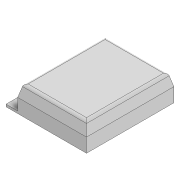
# Autodesk Inventor part: おもり
Saved by Autodesk Inventor 2020 (Build 240168000, 168)
## iProperties
Created: 2020-04-18
Part Number: おもり
Material: 一般
Document SubType Name: Modeling
Designer: highs
Density: 1 g/cm^3
Appearance: 既定
Author: highs
Autodesk Inventor part; units mm, degrees
ref_plane "YZ Plane" through (0, 0, 0) normal (1, 0, 0) x (0, 1, 0)
ref_plane "XZ Plane" through (0, 0, 0) normal (0, 1, 0) x (-1, 0, 0)
ref_plane "XY Plane" through (0, 0, 0) normal (0, 0, 1) x (1, 0, 0)
sketch "スケッチ1" plane through (0, 0, 0) normal (0, 0, 1) x (1, 0, 0)
  line L0 (0, 0) -> (138, 0)
  line L1 (138, 0) -> (138, 44)
  line L2 (138, 44) -> (20, 44)
  line L3 (20, 44) -> (20, 4)
  line L4 (20, 4) -> (0, 4)
  line L5 (0, 4) -> (0, 0)
  dimension "d0" = 20
  dimension "d1" = 4
  dimension "d2" = 40
  dimension "d3" = 118
  constraints: 12 end point, 4 perpendicular, 1 horizontal, 1 parallel
  measures "d0" distance of L3.end L4.end
  measures "d1" distance of L4.end L0.start
  measures "d2" distance of L2.end L3.end
  measures "d3" distance of L1.end L2.end
extrude "押し出し1" add sketch "スケッチ1" along normal blind 150
chamfer "面取り1" distance 5 distance2 20 1 edges at (20, 44, 75) measured on face at (98.6667, 44, 50)
chamfer "面取り2" distance 5 distance2 20 1 edges at (81.5, 44, 0) measured on face at (100.3333, 44, 50)
chamfer "面取り3" distance 5 distance2 20 1 edges at (138, 44, 77.5) measured on face at (100.3333, 44, 53.3333)
chamfer "面取り4" distance 5 distance2 20 1 edges at (79, 44, 150) measured on face at (97, 44, 101.6667)
fillet "フィレット1" radius 5 4 edges at (79, 44, 5) (25, 44, 75) (79, 44, 145) (133, 44, 75)
